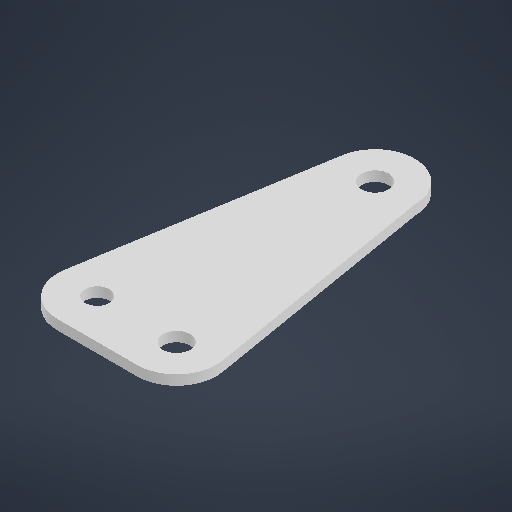
# Autodesk Inventor part: clampgeo
Saved by Autodesk Inventor 2025.2 (Build 292293000, 293)
## iProperties
Created: 2025-04-03
Part Number: clampgeo
Material: Generic
Document SubType Name: Modeling
Designer: Jahan
Density: 1 g/cm^3
Appearance: Default
Author: Jahan
Autodesk Inventor part; units mm, degrees
ref_plane "YZ Plane" through (0, 0, 0) normal (1, 0, 0) x (0, 1, 0)
ref_plane "XZ Plane" through (0, 0, 0) normal (0, 1, 0) x (-1, 0, 0)
ref_plane "XY Plane" through (0, 0, 0) normal (0, 0, 1) x (1, 0, 0)
sketch "Sketch1" plane through (0, 0, 0) normal (0, 1, 0) x (-1, 0, 0)
  circle A0 centre (0, 0) radius 2.1844
  line L0 (0, 0) -> (12.7, 0)
  circle A1 centre (12.7, 0) radius 1.9304
  line L1 (6.35, 0) -> (6.35, -38.1)
  circle A2 centre (6.35, -38.1) radius 2.1844
  circle A3 centre (12.7, 0) radius 6.35
  circle A4 centre (0, 0) radius 6.35
  circle A5 centre (6.35, -38.1) radius 6.35
  line L2 (18.9636, -1.0439) -> (12.6136, -39.1439)
  line L3 (-6.2612, -1.0583) -> (0, -38.1)
  line L4 (12.6136, 6.3494) -> (0.0003, 6.35)
  dimension "d0" = 4.3688
  dimension "d1" = 12.7
  dimension "d2" = 3.8608
  dimension "d3" = 38.1
  dimension "d4" = 4.3688
  dimension "d5" = 12.7
  dimension "d6" = 12.7
  constraints: 10 end point, 7 point on circle, 6 centre point, 6 coincident, 4 tangent, 1 horizontal, 1 midpoint, 1 vertical
  measures "d0" diameter of A0
  measures "d1" distance of L0.start L0.end
  measures "d2" diameter of A1
  measures "d3" distance of L1.start L1.end
  measures "d4" diameter of A2
  measures "d5" diameter of A3
  measures "d6" diameter of A5
extrude "Extrusion1" add sketch "Sketch1" along normal blind 1.5875
body "Solid1"
